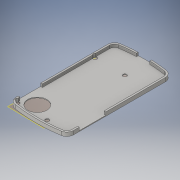
# Autodesk Inventor part: 32_Handycase_Nexus
Saved by Autodesk Inventor 2016 (Build 200138000, 138)
## iProperties
Created: 2016-09-23
Part Number: 32_Handycase_Nexus
Material: Generisch
Document SubType Name: Modeling
Designer: Bene
Density: 1 g/cm^3
Appearance: Vorgabe
Author: Bene
Autodesk Inventor part; units mm, degrees
ref_plane "YZ Plane" through (0, 0, 0) normal (1, 0, 0) x (0, 1, 0)
ref_plane "XZ Plane" through (0, 0, 0) normal (0, 1, 0) x (-1, 0, 0)
ref_plane "XY Plane" through (0, 0, 0) normal (0, 0, 1) x (1, 0, 0)
ref_plane "Arbeitsebene1" through (0.4278, -0.2817, 0) normal (0, 0, 1) x (0.9997967, -0.0201635, 0)
sketch "Skizze1" plane through (0.4278, -0.2817, 0) normal (0, 0, 1) x (0.9997967, -0.0201635, 0)
  arc A0 (45.5178, -51.289) -> (47.2273, -49.2152) centre (45.1652, -49.2568) ccw
  line L0 (47.2273, -49.2152) -> (44.7402, 74.105)
  arc A1 (44.7402, 74.105) -> (42.9485, 76.1081) centre (42.6781, 74.0634) ccw
  arc A2 (42.9485, 76.1081) -> (-16.8325, 74.9025) centre (17.0029, -120.1001) ccw
  arc A3 (-16.8325, 74.9025) -> (-18.542, 72.8287) centre (-16.4799, 72.8703) ccw
  line L1 (-18.542, 72.8287) -> (-16.0549, -50.4914)
  arc A4 (-16.0549, -50.4914) -> (-14.2632, -52.4946) centre (-13.9928, -50.4498) ccw
  arc A5 (-14.2632, -52.4946) -> (45.5178, -51.289) centre (11.6824, 143.7136) ccw
  line L2 (46.613, -43.5533) -> (-15.6694, -44.8094)
  line L3 (-15.6694, -44.8094) -> (-17.901, 65.8402)
  line L4 (-17.901, 65.8402) -> (44.3815, 67.0963)
  line L5 (44.3815, 67.0963) -> (46.613, -43.5533)
  circle A6 centre (35.5821, -49.45) radius 1
  circle A7 centre (15.5862, -49.8533) radius 2.25
  line L6 (51.7388, 74.2461) -> (54.2259, -49.074)
  arc A8 (46.7145, -58.1859) -> (54.2259, -49.074) centre (45.1652, -49.2568) ccw
  arc A9 (-15.1808, -59.4342) -> (46.7145, -58.1859) centre (11.6824, 143.7136) ccw
  arc A10 (-23.0535, -50.6326) -> (-15.1808, -59.4342) centre (-13.9928, -50.4498) ccw
  line L7 (-23.0535, -50.6326) -> (-25.5406, 72.6876)
  arc A11 (-18.0292, 81.7994) -> (-25.5406, 72.6876) centre (-16.4799, 72.8703) ccw
  arc A12 (43.8662, 83.0477) -> (-18.0292, 81.7994) centre (17.0029, -120.1001) ccw
  arc A13 (51.7388, 74.2461) -> (43.8662, 83.0477) centre (42.6781, 74.0634) ccw
  arc A14 (2.849, -38.7773) -> (-0.2109, -35.8384) centre (-0.1504, -38.8378) ccw construction
  line L8 (-0.2109, -35.8384) -> (-14.208, -36.1207) construction
  arc A15 (-17.2679, -33.1818) -> (-14.208, -36.1207) centre (-14.2685, -33.1213) ccw construction
  line L9 (-18.9358, 49.5185) -> (-17.2679, -33.1818) construction
  line L10 (-18.9358, 49.5185) -> (16.0684, 50.2244) construction
  line L11 (16.0684, 50.2244) -> (18.0689, -48.9725) construction
  line L12 (18.0689, -48.9725) -> (6.0601, -49.2147) construction
  arc A16 (3.0002, -46.2758) -> (6.0601, -49.2147) centre (5.9996, -46.2153) ccw construction
  line L13 (3.0002, -46.2758) -> (2.849, -38.7773) construction
  arc A17 (18.838, 55.1528) -> (17.9671, 55.2637) centre (18.0276, 52.2644) ccw construction
  line L14 (-21.0362, 54.4771) -> (17.9671, 55.2637) construction
  arc A18 (-21.0362, 54.4771) -> (-21.9019, 54.3312) centre (-20.9757, 51.4778) ccw construction
  arc A19 (-23.8642, 52.2881) -> (-21.9019, 54.3312) centre (-21.4857, 51.9676) ccw construction
  arc A20 (-23.8642, 52.2881) -> (-23.9751, 51.4173) centre (-20.9757, 51.4778) ccw construction
  line L15 (-21.8939, -51.7789) -> (-23.9751, 51.4173) construction
  arc A21 (-21.8939, -51.7789) -> (-21.7479, -52.6446) centre (-18.8945, -51.7184) ccw construction
  arc A22 (-19.7048, -54.6069) -> (-21.7479, -52.6446) centre (-19.3843, -52.2284) ccw construction
  arc A23 (-19.7048, -54.6069) -> (-18.834, -54.7178) centre (-18.8945, -51.7184) ccw construction
  line L16 (20.1693, -53.9312) -> (-18.834, -54.7178) construction
  arc A24 (20.1693, -53.9312) -> (21.035, -53.7852) centre (20.1089, -50.9318) ccw construction
  arc A25 (22.9973, -51.7422) -> (21.035, -53.7852) centre (20.6188, -51.4216) ccw construction
  arc A26 (22.9973, -51.7422) -> (23.1082, -50.8713) centre (20.1089, -50.9318) ccw construction
  line L17 (21.027, 52.3248) -> (23.1082, -50.8713) construction
  arc A27 (21.027, 52.3248) -> (20.8811, 53.1905) centre (18.0276, 52.2644) ccw construction
  arc A28 (18.838, 55.1528) -> (20.8811, 53.1905) centre (18.5175, 52.7743) ccw construction
  circle A29 centre (-4.5645, -42.5855) radius 5.1414 construction
  line L18 (-23.541, 72.7279) -> (-21.0539, -50.5922)
  arc A30 (-21.0539, -50.5922) -> (-14.9187, -57.4514) centre (-13.9928, -50.4498) ccw
  arc A31 (-14.9187, -57.4514) -> (46.3726, -56.2153) centre (11.6824, 143.7136) ccw
  arc A32 (46.3726, -56.2153) -> (52.2263, -49.1144) centre (45.1652, -49.2568) ccw
  line L19 (52.2263, -49.1144) -> (49.7392, 74.2058)
  arc A33 (49.7392, 74.2058) -> (43.604, 81.065) centre (42.6781, 74.0634) ccw
  arc A34 (43.604, 81.065) -> (-17.6873, 79.8289) centre (17.0029, -120.1001) ccw
  arc A35 (-17.6873, 79.8289) -> (-23.541, 72.7279) centre (-16.4799, 72.8703) ccw
  point P0 (-0.4334, 0.273)
  dimension "d0" = 7
  dimension "d3" = 2
  constraints: 66 point on circle, 40 end point, 36 centre point, 14 other
  measures "d0" distance between parallel lines of L0 L6
  measures "d3" distance between parallel lines of L7 L18
ref_plane "Arbeitsebene2" through (-16.0407, -51.963, 3.06) normal (0, 0, -1) x (-0.0201635, 0.9997967, 0)
extrude "Extrusion1" add sketch "Skizze1" along normal up to surface (3.06 mm away) contours A5 A4 L1 A3 A2 A1 L0 A0 | L2 L3 L4 L5 | A6 | A7 | L6 A8 A9 A10 L7 A11 A12 A13 | A35 A34 A33 L19 A32 A31 A30 L18
sketch "Skizze2" plane through (53.6532, -50.4391, 3.06) normal (0, 0, 1) x (1, 0, 0)
  arc A0 (-7.6936, -8.9586) -> (0, 0) centre (-9.0626, 0) ccw projected
  line L0 (0, 0) -> (0, 123.3452) projected
  arc A1 (0, 123.3452) -> (-7.6936, 132.3038) centre (-9.0626, 123.3452) ccw projected
  arc A2 (-7.6936, 132.3038) -> (-69.6015, 132.3038) centre (-38.6476, -70.2611) ccw projected
  arc A3 (-69.6015, 132.3038) -> (-77.2951, 123.3452) centre (-68.2326, 123.3452) ccw projected
  line L1 (-77.2951, 123.3452) -> (-77.2951, 0) projected
  arc A4 (-77.2951, 0) -> (-69.6015, -8.9586) centre (-68.2326, 0) ccw projected
  arc A5 (-69.6015, -8.9586) -> (-7.6936, -8.9586) centre (-38.6476, 193.6063) ccw projected
  arc A6 (-8.041, 130.0302) -> (-69.2541, 130.0302) centre (-38.6476, -70.2611) ccw
  arc A7 (-2.3, 123.3452) -> (-8.041, 130.0302) centre (-9.0626, 123.3452) ccw
  line L2 (-2.3, 123.3452) -> (-2.3, 0)
  arc A8 (-8.041, -6.685) -> (-2.3, 0) centre (-9.0626, 0) ccw
  arc A9 (-69.2541, -6.685) -> (-8.041, -6.685) centre (-38.6476, 193.6063) ccw
  arc A10 (-74.9951, 0) -> (-69.2541, -6.685) centre (-68.2326, 0) ccw
  line L3 (-74.9951, 0) -> (-74.9951, 123.3452)
  arc A11 (-69.2541, 130.0302) -> (-74.9951, 123.3452) centre (-68.2326, 123.3452) ccw
  point P0 (-53.6532, 50.4391)
  dimension "d4" = 2.3
  constraints: 12 point on circle, 6 centre point, 4 end point, 7 other
  measures "d4" radial gap between concentric circles of A2 A6
extrude "Extrusion2" add sketch "Skizze2" along normal blind 4
sketch "Skizze3" plane through (0.4278, -0.2817, 0) normal (0, 0, -1) x (-0.9997967, 0.0201635, 0)
  circle A0 centre (-15.5862, -49.8533) radius 2.25 projected
  arc A1 (-20.8811, 53.1905) -> (-18.838, 55.1528) centre (-18.5175, 52.7743) ccw projected
  arc A2 (21.9019, 54.3312) -> (23.8642, 52.2881) centre (21.4857, 51.9676) ccw projected
  arc A3 (21.7479, -52.6446) -> (19.7048, -54.6069) centre (19.3843, -52.2284) ccw projected
  arc A4 (-21.035, -53.7852) -> (-22.9973, -51.7422) centre (-20.6188, -51.4216) ccw projected
  ellipse E0 centre (4.1989, -40.6786) end of major axis (4.456, -27.9312) minor radius 12.7499 projected
  circle A5 centre (19.3843, -52.2284) radius 2.5
  circle A6 centre (-20.6188, -51.4216) radius 2.5
  circle A7 centre (-18.5175, 52.7743) radius 2.5
  circle A8 centre (21.4857, 51.9676) radius 2.5
  point P0 (0.4334, 0.273)
  dimension "d7" = 5
  dimension "d8" = 5
  dimension "d9" = 5
  dimension "d10" = 5
  constraints: 4 centre point, 4 coincident, 1 other
  measures "d7" diameter of A5
  measures "d8" diameter of A6
  measures "d9" diameter of A7
  measures "d10" diameter of A8
extrude "Extrusion3" cut sketch "Skizze3" against normal through all contours E0 | A5 | A6 | A7 | A8
sketch "Skizze4" plane through (53.6532, -50.4391, 7.06) normal (0, 0, 1) x (1, 0, 0)
  arc A0 (-74.9951, 104.6606) -> (-74.9951, 100.4348) centre (-73.6588, 102.5477) ccw projected
  line L0 (-74.9951, 104.6606) -> (-74.9951, 123.3452) projected
  arc A1 (-69.2541, 130.0302) -> (-74.9951, 123.3452) centre (-68.2326, 123.3452) ccw projected
  arc A2 (-8.041, 130.0302) -> (-69.2541, 130.0302) centre (-38.6476, -70.2611) ccw projected
  arc A3 (-2.3, 123.3452) -> (-8.041, 130.0302) centre (-9.0626, 123.3452) ccw projected
  line L1 (-2.3, 123.3452) -> (-2.3, 0) projected
  arc A4 (-8.041, -6.685) -> (-2.3, 0) centre (-9.0626, 0) ccw projected
  arc A5 (-69.2541, -6.685) -> (-8.041, -6.685) centre (-38.6476, 193.6063) ccw projected
  arc A6 (-73.5584, -4.1674) -> (-69.2541, -6.685) centre (-68.2326, 0) ccw projected
  arc A7 (-74.9951, 0.4434) -> (-73.5584, -4.1674) centre (-73.6588, -1.6695) ccw projected
  arc A8 (-77.2951, 0) -> (-69.6015, -8.9586) centre (-68.2326, 0) ccw projected
  arc A9 (-69.6015, -8.9586) -> (-7.6936, -8.9586) centre (-38.6476, 193.6063) ccw projected
  arc A10 (-7.6936, -8.9586) -> (0, 0) centre (-9.0626, 0) ccw projected
  line L2 (0, 0) -> (0, 123.3452) projected
  arc A11 (0, 123.3452) -> (-7.6936, 132.3038) centre (-9.0626, 123.3452) ccw projected
  arc A12 (-7.6936, 132.3038) -> (-69.6015, 132.3038) centre (-38.6476, -70.2611) ccw projected
  arc A13 (-69.6015, 132.3038) -> (-77.2951, 123.3452) centre (-68.2326, 123.3452) ccw projected
  line L3 (-77.2951, 123.3452) -> (-77.2951, 0) projected
  line L4 (-74.9951, 0.4434) -> (-74.9951, 100.4348) projected
  line L5 (-81.9531, 2.9217) -> (-72.1543, 2.9217)
  line L6 (-72.1543, 2.9217) -> (-72.1543, 33.2257)
  line L7 (-72.1543, 33.2257) -> (-81.9531, 33.2257)
  line L8 (-81.9531, 33.2257) -> (-81.9531, 2.9217)
  line L9 (-81.9531, 2.9217) -> (-72.1543, 33.2257) construction
  line L10 (-72.1543, 2.9217) -> (-81.9531, 33.2257) construction
  line L11 (-8.5397, 7.6973) -> (3.9397, 7.6973)
  line L12 (3.9397, 7.6973) -> (3.9397, 43.3206)
  line L13 (3.9397, 43.3206) -> (-8.5397, 43.3206)
  line L14 (-8.5397, 43.3206) -> (-8.5397, 7.6973)
  line L15 (-8.5397, 7.6973) -> (3.9397, 43.3206) construction
  line L16 (3.9397, 7.6973) -> (-8.5397, 43.3206) construction
  line L17 (-47.6229, 127.8641) -> (-29.6723, 127.8641)
  line L18 (-29.6723, 127.8641) -> (-29.6723, 136.8462)
  line L19 (-29.6723, 136.8462) -> (-47.6229, 136.8462)
  line L20 (-47.6229, 136.8462) -> (-47.6229, 127.8641)
  line L21 (-47.6229, 127.8641) -> (-29.6723, 136.8462) construction
  line L22 (-29.6723, 127.8641) -> (-47.6229, 136.8462) construction
  point P0 (-53.6532, 50.4391)
  point P1 (-77.0537, 18.0737)
  point P2 (-2.3, 25.5089)
  point P3 (-38.6476, 132.3552)
  constraints: 36 end point, 6 midpoint, 6 parallel, 3 horizontal, 3 perpendicular, 1 point on circle, 1 point on line
extrude "Extrusion4" cut sketch "Skizze4" against normal up to surface (4 mm away) contours L7 L6 L5 L4 | L4 L5 L3 L7 | L3 L5 L8 L7 | L20 A12 L18 A2 | A2 L18 L17 L20 | L20 L19 L18 A12 | L13 L2 L11 L1 | L1 L11 L14 L13 | L13 L12 L11 L2
sketch "Skizze5" plane through (0.4278, -0.2817, 0) normal (0, 0, -1) x (-0.9997967, 0.0201635, 0)
  circle A0 centre (21.4857, 51.9676) radius 2.5 projected
  circle A1 centre (-20.6188, -51.4216) radius 2.5 projected
  circle A2 centre (19.3843, -52.2284) radius 2.5 projected
  circle A3 centre (-18.5175, 52.7743) radius 2.5 projected
  ellipse E0 centre (4.1989, -40.6786) end of major axis (3.9418, -53.426) minor radius 12.7499 projected
  line L0 (-51.7388, 74.2461) -> (-54.2259, -49.074) projected
  arc A4 (-54.2259, -49.074) -> (-46.7145, -58.1859) centre (-45.1652, -49.2568) ccw projected
  arc A5 (-46.7145, -58.1859) -> (15.1808, -59.4342) centre (-11.6824, 143.7136) ccw projected
  arc A6 (15.1808, -59.4342) -> (23.0535, -50.6326) centre (13.9928, -50.4498) ccw projected
  line L1 (23.0535, -50.6326) -> (25.5406, 72.6876) projected
  arc A7 (25.5406, 72.6876) -> (18.0292, 81.7994) centre (16.4799, 72.8703) ccw projected
  arc A8 (18.0292, 81.7994) -> (-43.8662, 83.0477) centre (-17.0029, -120.1001) ccw projected
  arc A9 (-43.8662, 83.0477) -> (-51.7388, 74.2461) centre (-42.6781, 74.0634) ccw projected
  point P0 (0.4334, 0.273)
  constraints: 1 other
extrude "Extrusion5" cut sketch "Skizze5" against normal blind 2
